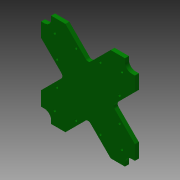
# Autodesk Inventor part: bed2
Saved by Autodesk Inventor 2014 (Build 180170000, 170)
## iProperties
Created: 2015-06-29
Part Number: bed2
Material: Generic
Document SubType Name: Modeling
Designer: cruiser
Density: 1 g/cm^3
Appearance: Default
Author: cruiser
Autodesk Inventor part; units mm, degrees
ref_plane "YZ Plane" through (0, 0, 0) normal (1, 0, 0) x (0, 1, 0)
ref_plane "XZ Plane" through (0, 0, 0) normal (0, 1, 0) x (-1, 0, 0)
ref_plane "XY Plane" through (0, 0, 0) normal (0, 0, 1) x (1, 0, 0)
sketch "Sketch1" plane through (0, 0, 0) normal (0, 1, 0) x (-1, 0, 0)
  line L0 (70.5, -70.5) -> (-70.5, -70.5)
  line L1 (-70.5, -70.5) -> (-70.5, 70.5)
  line L2 (-70.5, 70.5) -> (70.5, 70.5)
  line L3 (70.5, 70.5) -> (70.5, -70.5)
  line L4 (70.5, -70.5) -> (-70.5, 70.5) construction
  line L5 (-70.5, -70.5) -> (70.5, 70.5) construction
  point P0 (0, 0)
  dimension "d0" = 141
  dimension "d1" = 141
  constraints: 12 end point, 2 midpoint, 2 parallel, 1 horizontal, 1 perpendicular
  measures "d0" distance of L1.end L2.end
  measures "d1" distance of L0.end L1.end
extrude "Extrusion1" add sketch "Sketch1" along normal blind 5.88
sketch "Sketch2" plane through (0, 5.88, 0) normal (0, 1, 0) x (1, 0, 0)
  line L0 (75.5, -75.5) -> (-75.5, -75.5)
  line L1 (-75.5, -75.5) -> (-75.5, 75.5)
  line L2 (-75.5, 75.5) -> (75.5, 75.5)
  line L3 (75.5, 75.5) -> (75.5, -75.5)
  line L4 (75.5, -75.5) -> (-75.5, 75.5) construction
  line L5 (-75.5, -75.5) -> (75.5, 75.5) construction
  line L6 (-95.5, 95.5) -> (-55.5, 95.5)
  line L7 (-55.5, 95.5) -> (-55.5, 65.5)
  line L8 (-65.5, 55.5) -> (-95.5, 55.5)
  line L9 (-95.5, 55.5) -> (-95.5, 95.5)
  line L10 (-95.5, 95.5) -> (-55.5, 55.5) construction
  line L11 (-55.5, 95.5) -> (-95.5, 55.5) construction
  arc A0 (-65.5, 55.5) -> (-55.5, 65.5) centre (-65.5, 65.5) ccw
  line L12 (-95.5, -95.5) -> (-55.5, -95.5)
  line L13 (-55.5, -95.5) -> (-55.5, -65.5)
  line L14 (-65.5, -55.5) -> (-95.5, -55.5)
  line L15 (-95.5, -55.5) -> (-95.5, -95.5)
  line L16 (-95.5, -95.5) -> (-55.5, -55.5) construction
  line L17 (-55.5, -95.5) -> (-95.5, -55.5) construction
  arc A1 (-55.5, -65.5) -> (-65.5, -55.5) centre (-65.5, -65.5) ccw
  line L18 (0, 0) -> (0, -75.5)
  line L19 (75.5, -75.5) -> (75.5, 75.5)
  line L20 (95.5, 95.5) -> (55.5, 95.5)
  line L21 (55.5, 95.5) -> (55.5, 65.5)
  line L22 (65.5, 55.5) -> (95.5, 55.5)
  line L23 (95.5, 55.5) -> (95.5, 95.5)
  line L24 (95.5, 95.5) -> (55.5, 55.5) construction
  line L25 (55.5, 95.5) -> (95.5, 55.5) construction
  arc A2 (55.5, 65.5) -> (65.5, 55.5) centre (65.5, 65.5) ccw
  line L26 (95.5, -95.5) -> (55.5, -95.5)
  line L27 (55.5, -95.5) -> (55.5, -65.5)
  line L28 (65.5, -55.5) -> (95.5, -55.5)
  line L29 (95.5, -55.5) -> (95.5, -95.5)
  line L30 (95.5, -95.5) -> (55.5, -55.5) construction
  line L31 (55.5, -95.5) -> (95.5, -55.5) construction
  arc A3 (65.5, -55.5) -> (55.5, -65.5) centre (65.5, -65.5) ccw
  line L32 (70.5, 70.5) -> (70.5, -70.5)
  dimension "d4" = 151
  dimension "d5" = 151
  dimension "d6" = 40
  dimension "d7" = 40
  dimension "d8" = 10
  dimension "d11" = 40
  dimension "d12" = 40
  dimension "d13" = 10
  constraints: 66 end point, 14 symmetric about line, 11 midpoint, 8 point on circle, 8 point on line, 6 parallel, 4 centre point, 4 tangent, 3 horizontal, 3 perpendicular, 2 other
  measures "d4" distance of L1.end L2.end
  measures "d5" distance of L0.end L1.end
  measures "d6" distance of L10.end L8.end
  measures "d7" distance of L6.end L10.end
  measures "d8" radius of A0
  measures "d11" distance of L14.end L16.end
  measures "d12" distance of L16.end L12.end
  measures "d13" radius of A1
extrude "Extrusion2" cut sketch "Sketch2" against normal blind 5.88 contours L3 L28 L29 L26 L27 L0 | L0 L27 A3 L28 L3 | L22 A2 L21 L2 L3 | L3 L2 L21 L20 L23 L22 | L13 L12 L15 L14 L1 L0 | L0 L1 L14 A1 L13 | L7 A0 L8 L1 L2 | L2 L1 L8 L9 L6 L7
sketch "Sketch3" plane through (0, 0, 0) normal (0, -1, 0) x (1, 0, 0)
  line L0 (-55.5, 70.5) -> (-55.5, 65.5) projected
  arc A0 (-65.5, 55.5) -> (-55.5, 65.5) centre (-65.5, 65.5) ccw projected
  line L1 (-65.5, 55.5) -> (-70.5, 55.5) projected
  line L2 (-70.5, 55.5) -> (-70.5, -70.5) projected
  line L3 (-70.5, -70.5) -> (70.5, -70.5) projected
  line L4 (70.5, -70.5) -> (70.5, 70.5) projected
  line L5 (70.5, 70.5) -> (-55.5, 70.5) projected
  point P0 (0, 0)
  point P1 (-60.5, 56.8397)
  constraints: 2 other
extrude "Extrusion3" add sketch "Sketch3" along normal blind 3.15 separate body
sketch "Sketch18" plane through (0, -3.15, 0) normal (0, -1, 0) x (1, 0, 0)
  line L0 (-55.5, 70.5) -> (-55.5, 65.5) projected
  arc A0 (-65.5, 55.5) -> (-55.5, 65.5) centre (-65.5, 65.5) ccw projected
  line L1 (-65.5, 55.5) -> (-70.5, 55.5) projected
  line L2 (-70.5, 55.5) -> (-70.5, -70.5) projected
  line L3 (-70.5, -70.5) -> (70.5, -70.5) projected
  line L4 (70.5, -70.5) -> (70.5, 70.5) projected
  line L5 (70.5, 70.5) -> (-55.5, 70.5) projected
  point P0 (0, 0)
extrude "Extrusion17" add sketch "Sketch18" along normal blind 3.15 separate body
sketch "Sketch5" plane through (0, 5.88, 0) normal (0, 1, 0) x (1, 0, 0)
  line L0 (-55.5, -65.5) -> (-55.5, -70.5) projected
  line L1 (-55.5, -70.5) -> (70.5, -70.5) projected
  line L2 (70.5, -70.5) -> (70.5, 70.5) projected
  line L3 (70.5, 70.5) -> (-70.5, 70.5) projected
  line L4 (-70.5, 70.5) -> (-70.5, -55.5) projected
  line L5 (-70.5, -55.5) -> (-65.5, -55.5) projected
  arc A0 (-55.5, -65.5) -> (-65.5, -55.5) centre (-65.5, -65.5) ccw projected
  point P0 (0, 0)
  point P1 (-60.5, -56.8397)
  constraints: 2 other
extrude "Extrusion5" add sketch "Sketch5" along normal blind 5.88 separate body
sketch "Sketch14" plane through (0, 11.76, 0) normal (0, 1, 0) x (1, 0, 0)
  line L0 (70.5, 70.5) -> (-70.5, 70.5) projected
  line L1 (-70.5, 70.5) -> (-70.5, -55.5) projected
  circle A0 centre (-40.5, 40.5) radius 2
  line L2 (0, 0) -> (10.755, 0)
  line L3 (10.755, 0) -> (10.755, -13.1372)
  line L4 (10.755, -13.1372) -> (0, -13.1372)
  line L5 (0, -13.1372) -> (0, 0)
  circle A1 centre (-50.5, 50.5) radius 1.575
  circle A2 centre (40.5, 40.5) radius 2
  circle A3 centre (50.5, 50.5) radius 1.575
  circle A4 centre (-40.5, -40.5) radius 2
  circle A5 centre (-50.5, -50.5) radius 1.575
  circle A6 centre (40.5, -40.5) radius 2
  circle A7 centre (50.5, -50.5) radius 1.575
  dimension "d87" = 4
  dimension "d88" = 30
  dimension "d89" = 30
  dimension "d90" = 3.15
  dimension "d91" = 20
  dimension "d92" = 20
  constraints: 8 centre point, 8 end point, 6 symmetric about line, 2 parallel, 1 horizontal, 1 perpendicular, 6 other
  measures "d87" diameter of A0
  measures "d88" distance from line of L1 A0.centre
  measures "d89" distance from line of L0 A0.centre
  measures "d90" diameter of A1
  measures "d91" distance from line of L1 A1.centre
  measures "d92" distance from line of L0 A1.centre
extrude "Extrusion14" cut sketch "Sketch14" against normal up to next contours A0 | A1 | A2 | A3 | A4 | A5 | A6 | A7 bodies 4
sketch "Sketch12" plane through (0, 11.76, 0) normal (0, 1, 0) x (1, 0, 0)
  line L0 (70.5, 70.5) -> (-70.5, 70.5) projected
  line L1 (-70.5, 70.5) -> (-70.5, -55.5) projected
  line L2 (0, 20) -> (-50.5, 70.5)
  line L3 (-50.5, 70.5) -> (0, 121)
  line L4 (0, 121) -> (50.5, 70.5)
  line L5 (50.5, 70.5) -> (0, 20)
  line L6 (0, 0) -> (-70.5, 0)
  line L7 (0, 0) -> (0, 70.5)
  line L8 (-20, 0) -> (-70.5, -50.5)
  line L9 (-70.5, -50.5) -> (-121, 0)
  line L10 (-121, 0) -> (-70.5, 50.5)
  line L11 (-70.5, 50.5) -> (-20, 0)
  line L12 (0, -20) -> (-50.5, -70.5)
  line L13 (-50.5, -70.5) -> (0, -121)
  line L14 (0, -121) -> (50.5, -70.5)
  line L15 (50.5, -70.5) -> (0, -20)
  line L16 (20, 0) -> (70.5, -50.5)
  line L17 (70.5, -50.5) -> (121, 0)
  line L18 (121, 0) -> (70.5, 50.5)
  line L19 (70.5, 50.5) -> (20, 0)
  point P0 (-70.5, 0)
  dimension "d76" = 20
  dimension "d77" = 20
  constraints: 36 end point, 8 symmetric about line, 3 point on line, 2 perpendicular, 1 coincident, 1 midpoint, 18 other
  measures "d76" distance of L6.start L2.start
  measures "d77" distance of L6.start L8.start
extrude "Extrusion12" cut sketch "Sketch12" against normal up to next contours L5 L7 L0 | L0 L3 L4 | L7 L2 L0 | L8 L1 L6 | L6 L1 L11 | L1 L9 L10 | L15 L14 L13 L12 | L19 L18 L17 L16 bodies 4
sketch "Sketch15" plane through (0, 5.88, 0) normal (0, 1, 0) x (1, 0, 0)
  line L0 (70.5, 70.5) -> (-70.5, 70.5) projected
  line L1 (-70.5, 70.5) -> (-70.5, -55.5) projected
  circle A0 centre (-50.5, 50.5) radius 2
  circle A1 centre (-40.5, 40.5) radius 4
  line L2 (0, 0) -> (13.8071, 0)
  line L3 (13.8071, 0) -> (13.8071, -11.5249)
  line L4 (13.8071, -11.5249) -> (0, -11.5249)
  line L5 (0, -11.5249) -> (0, 0)
  circle A2 centre (50.5, 50.5) radius 2
  circle A3 centre (40.5, 40.5) radius 4
  circle A4 centre (-50.5, -50.5) radius 2
  circle A5 centre (-40.5, -40.5) radius 4
  circle A6 centre (40.5, -40.5) radius 4
  circle A7 centre (50.5, -50.5) radius 2
  point P0 (-70.5, -55.5)
  point P1 (-60.5, -56.8397)
  dimension "d95" = 8
  dimension "d96" = 4
  dimension "d97" = 30
  dimension "d98" = 30
  dimension "d99" = 20
  dimension "d100" = 20
  constraints: 8 centre point, 8 end point, 6 symmetric about line, 2 parallel, 1 horizontal, 1 perpendicular, 7 other
  measures "d95" diameter of A1
  measures "d96" diameter of A0
  measures "d98" distance from line of L0 A1.centre
  measures "d100" distance from line of L0 A0.centre
extrude "Extrusion15" cut sketch "Sketch15" against normal up to next contours A0 | A2 | A4 | A7 bodies 1
sketch "Sketch9" plane through (0, 5.88, 0) normal (0, 1, 0) x (1, 0, 0)
  line L0 (70.5, -70.5) -> (70.5, 70.5) projected
  line L1 (-70.5, -55.5) -> (-65.5, -55.5) projected
  circle A0 centre (47, 18.28) radius 2
  line L2 (70.5, 30) -> (0, 30)
  line L3 (0, 0) -> (70.5, 70.5)
  circle A1 centre (18.28, 47) radius 2
  dimension "d58" = 4
  dimension "d59" = 47
  dimension "d60" = 30
  dimension "d61" = 11.72
  constraints: 4 end point, 2 centre point, 1 parallel, 1 point on line, 1 symmetric about line, 1 other
  measures "d58" diameter of A0
  measures "d59" horizontal distance of L3.start A0.centre
  measures "d60" distance from line of L3.start L2
  measures "d61" distance from line of L2 A0.centre
extrude "Extrusion9" cut sketch "Sketch9" against normal up to next contours A0 | A1 bodies 1
sketch "Sketch16" plane through (0, 0, 0) normal (0, 1, 0) x (1, 0, 0)
  line L0 (-70.5, 70.5) -> (70.5, 70.5) projected
  circle A0 centre (-50.5, 50.5) radius 4
  line L1 (0, 0) -> (13.4297, 0)
  line L2 (13.4297, 0) -> (13.4297, -12.6623)
  line L3 (13.4297, -12.6623) -> (0, -12.6623)
  line L4 (0, -12.6623) -> (0, 0)
  circle A1 centre (50.5, 50.5) radius 4
  circle A2 centre (-50.5, -50.5) radius 4
  circle A3 centre (50.5, -50.5) radius 4
  point P0 (-70.5, -55.5)
  dimension "d103" = 8
  dimension "d104" = 20
  dimension "d105" = 20
  constraints: 8 end point, 4 centre point, 3 symmetric about line, 2 parallel, 1 horizontal, 1 perpendicular, 4 other
  measures "d103" diameter of A0
  measures "d105" distance from line of L0 A0.centre
extrude "Extrusion16" cut sketch "Sketch16" against normal up to next contours A0 | A1 | A2 | A3 bodies 2
sketch "Sketch19" plane through (0, 11.76, 0) normal (0, 1, 0) x (1, 0, 0)
  line L0 (0, 20) -> (-50.5, 70.5) projected
  line L1 (50.5, 70.5) -> (0, 20) projected
  line L2 (0, 12.9289) -> (-28.2843, 41.2132)
  line L3 (-28.2843, 41.2132) -> (0, 69.4975)
  line L4 (0, 69.4975) -> (28.2843, 41.2132)
  line L5 (28.2843, 41.2132) -> (0, 12.9289)
  line L6 (-12.9289, 0) -> (-41.2132, -28.2843)
  line L7 (-41.2132, -28.2843) -> (-69.4975, 0)
  line L8 (-69.4975, 0) -> (-41.2132, 28.2843)
  line L9 (-41.2132, 28.2843) -> (-12.9289, 0)
  line L10 (0, -12.9289) -> (28.2843, -41.2132)
  line L11 (28.2843, -41.2132) -> (0, -69.4975)
  line L12 (0, -69.4975) -> (-28.2843, -41.2132)
  line L13 (-28.2843, -41.2132) -> (0, -12.9289)
  line L14 (12.9289, 0) -> (41.2132, 28.2843)
  line L15 (41.2132, 28.2843) -> (69.4975, 0)
  line L16 (69.4975, 0) -> (41.2132, -28.2843)
  line L17 (41.2132, -28.2843) -> (12.9289, 0)
  line L18 (-28.2843, 41.2132) -> (28.2843, 41.2132)
  line L19 (28.2843, 41.2132) -> (28.2843, 81.2132)
  line L20 (28.2843, 81.2132) -> (-28.2843, 81.2132)
  line L21 (-28.2843, 81.2132) -> (-28.2843, 41.2132)
  line L22 (-41.2132, -28.2843) -> (-41.2132, 28.2843)
  line L23 (-41.2132, 28.2843) -> (-81.2132, 28.2843)
  line L24 (-81.2132, 28.2843) -> (-81.2132, -28.2843)
  line L25 (-81.2132, -28.2843) -> (-41.2132, -28.2843)
  line L26 (28.2843, -41.2132) -> (-28.2843, -41.2132)
  line L27 (-28.2843, -41.2132) -> (-28.2843, -81.2132)
  line L28 (-28.2843, -81.2132) -> (28.2843, -81.2132)
  line L29 (28.2843, -81.2132) -> (28.2843, -41.2132)
  line L30 (41.2132, 28.2843) -> (41.2132, -28.2843)
  line L31 (41.2132, -28.2843) -> (81.2132, -28.2843)
  line L32 (81.2132, -28.2843) -> (81.2132, 28.2843)
  line L33 (81.2132, 28.2843) -> (41.2132, 28.2843)
  point P0 (0, 0)
  dimension "d110" = 5
  dimension "d111" = 5
  dimension "d112" = 40
  dimension "d113" = 40
  dimension "d116" = 360
  dimension "d127" = 40
  dimension "d130" = 360
  constraints: 64 end point, 5 parallel, 2 perpendicular, 66 other
  measures "d110" distance between parallel lines of L1 L5
  measures "d111" distance between parallel lines of L2 L0
  measures "d112" distance of L2.end L3.end
  measures "d113" distance between parallel lines of L3 L5
  measures "d127" distance of L4.end L19.end
extrude "Extrusion18" cut sketch "Sketch19" against normal up to next bodies 4
sketch "Sketch20" plane through (0, 5.88, 0) normal (0, 1, 0) x (1, 0, 0)
  line L0 (70.5, 70.5) -> (-70.5, 70.5) projected
  line L1 (0, 36.5) -> (-34, 70.5)
  line L2 (-34, 70.5) -> (0, 104.5)
  line L3 (0, 104.5) -> (34, 70.5)
  line L4 (34, 70.5) -> (0, 36.5)
  line L5 (-36.5, 0) -> (-70.5, -34)
  line L6 (-70.5, -34) -> (-104.5, 0)
  line L7 (-104.5, 0) -> (-70.5, 34)
  line L8 (-70.5, 34) -> (-36.5, 0)
  line L9 (0, -36.5) -> (34, -70.5)
  line L10 (34, -70.5) -> (0, -104.5)
  line L11 (0, -104.5) -> (-34, -70.5)
  line L12 (-34, -70.5) -> (0, -36.5)
  line L13 (36.5, 0) -> (70.5, 34)
  line L14 (70.5, 34) -> (104.5, 0)
  line L15 (104.5, 0) -> (70.5, -34)
  line L16 (70.5, -34) -> (36.5, 0)
  point P0 (0, 0)
  point P1 (0, 70.5)
  point P2 (0, 0)
  point P3 (-70.5, 0)
  point P4 (0, 0)
  point P5 (0, -70.5)
  point P6 (0, 0)
  point P7 (70.5, 0)
  dimension "d120" = 34
  dimension "d123" = 360
  constraints: 32 end point, 2 coincident, 1 midpoint, 1 point on line, 48 other
  measures "d120" distance from line of L0 L1.start
extrude "Extrusion19" cut sketch "Sketch20" against normal up to next bodies 1
sketch "Sketch23" plane through (0, 11.76, 0) normal (0, 1, 0) x (1, 0, 0)
  line L0 (-75.5, -75.5) -> (75.5, -75.5)
  line L1 (75.5, -75.5) -> (75.5, 75.5)
  line L2 (75.5, 75.5) -> (-75.5, 75.5)
  line L3 (-75.5, 75.5) -> (-75.5, -75.5)
  line L4 (-75.5, -75.5) -> (75.5, 75.5) construction
  line L5 (75.5, -75.5) -> (-75.5, 75.5) construction
  line L6 (-70.5, 55.5) -> (-95.5, 55.5)
  line L7 (-95.5, 55.5) -> (-95.5, 95.5)
  line L8 (-95.5, 95.5) -> (-55.5, 95.5)
  line L9 (-55.5, 95.5) -> (-55.5, 70.5)
  line L10 (-55.5, 55.5) -> (-95.5, 95.5) construction
  line L11 (-95.5, 55.5) -> (-55.5, 95.5) construction
  arc A0 (-70.5, 55.5) -> (-55.5, 70.5) centre (-70.5, 70.5) ccw
  line L12 (-55.5, -70.5) -> (-55.5, -95.5)
  line L13 (-55.5, -95.5) -> (-95.5, -95.5)
  line L14 (-95.5, -95.5) -> (-95.5, -55.5)
  line L15 (-95.5, -55.5) -> (-70.5, -55.5)
  line L16 (-55.5, -55.5) -> (-95.5, -95.5) construction
  line L17 (-55.5, -95.5) -> (-95.5, -55.5) construction
  arc A1 (-55.5, -70.5) -> (-70.5, -55.5) centre (-70.5, -70.5) ccw
  line L18 (70.5, -55.5) -> (95.5, -55.5)
  line L19 (95.5, -55.5) -> (95.5, -95.5)
  line L20 (95.5, -95.5) -> (55.5, -95.5)
  line L21 (55.5, -95.5) -> (55.5, -70.5)
  line L22 (55.5, -55.5) -> (95.5, -95.5) construction
  line L23 (95.5, -55.5) -> (55.5, -95.5) construction
  arc A2 (70.5, -55.5) -> (55.5, -70.5) centre (70.5, -70.5) ccw
  line L24 (55.5, 70.5) -> (55.5, 95.5)
  line L25 (55.5, 95.5) -> (95.5, 95.5)
  line L26 (95.5, 95.5) -> (95.5, 55.5)
  line L27 (95.5, 55.5) -> (70.5, 55.5)
  line L28 (55.5, 55.5) -> (95.5, 95.5) construction
  line L29 (55.5, 95.5) -> (95.5, 55.5) construction
  arc A3 (55.5, 70.5) -> (70.5, 55.5) centre (70.5, 70.5) ccw
  point P0 (-70.5, 70.5)
  point P1 (-70.5, 50.5)
  point P2 (0, 0)
  point P3 (-70.5, -70.5)
  point P4 (-50.5, -70.5)
  point P5 (-75.5, -75.5)
  point P6 (70.5, -70.5)
  point P7 (70.5, -50.5)
  point P8 (75.5, -75.5)
  point P9 (70.5, 70.5)
  point P10 (50.5, 70.5)
  point P11 (75.5, 75.5)
  dimension "d135" = 151
  dimension "d136" = 151
  dimension "d137" = 40
  dimension "d138" = 40
  dimension "d139" = 15
  dimension "d142" = 360
  constraints: 60 end point, 10 midpoint, 8 point on circle, 8 point on line, 4 centre point, 4 parallel, 2 horizontal, 2 perpendicular, 2 tangent, 69 other
  measures "d135" distance of L2.end L1.end
  measures "d136" distance of L1.end L0.end
  measures "d137" distance of L7.end L8.end
  measures "d138" distance of L6.end L7.end
  measures "d139" radius of A0
extrude "Extrusion20" cut sketch "Sketch23" against normal up to next contours L21 A2 L18 L1 L0 | L0 L1 L18 L19 L20 L21 | L6 L7 L8 L9 L2 L3 | L3 L2 L9 A0 L6 | L27 A3 L24 L2 L1 | L1 L2 L24 L25 L26 L27 bodies 4
fillet "Fillet1" radius 5 8 edges at (36.5, 2.94, 0) (0, 2.94, -36.5) (-36.5, 2.94, 0) (0, 2.94, 36.5) (0, 8.82, -12.9289) (12.9289, 8.82, 0) (0, 8.82, 12.9289) (-12.9289, 8.82, 0)
pattern_circular "Circular Pattern1" count 4 over 360 about axis through (0, -10, 0) along (0, 1, 0) of "Extrusion9" bodies 1
equation "\"d0\" = bed_x"
equation "\"d1\" = bed_y"
equation "\"d2\" = t_wall"
equation "\"d4\" = reservoir_x"
equation "\"d5\" = reservoir_y"
equation "\"d9\" = t_wall"
equation "\"d14\" = clear_acrylic"
equation "\"d108\" = thin_acrylic"
equation "\"d18\" = t_carrier"
equation "\"d87\" = brass_insert_drill"
equation "\"d88\" = spring_border"
equation "\"d89\" = spring_border"
equation "\"d90\" = m3_diameter"
equation "\"d91\" = bed_clamp_border"
equation "\"d92\" = bed_clamp_border"
equation "\"d96\" = brass_insert_drill"
equation "\"d97\" = spring_border"
equation "\"d98\" = spring_border"
equation "\"d99\" = bed_clamp_border"
equation "\"d100\" = bed_clamp_border"
equation "\"d101\" = t_carrier"
equation "\"d58\" = brass_insert_drill"
equation "\"d59\" = end_stop_offset_x"
equation "\"d60\" = 0.5 * crane_y"
equation "\"d61\" = thumb_nut_offset_y"
equation "\"d104\" = bed_clamp_border"
equation "\"d105\" = bed_clamp_border"
equation "\"d106\" = t_carrier"
equation "\"thick_acrylic\" = 5.88"
equation "\"thin_acrylic\" = 3.15"
equation "\"clear_acrylic\" = 3.15"
equation "\"wood_thickness\" = 6.72"
equation "\"m3_diameter\" = 3.15"
equation "\"m4_diameter\" = 4.2"
equation "\"m5_diameter\" = 5.25"
equation "\"brass_insert_drill\" = 4"
equation "\"stepper_screw_space\" = 35"
equation "\"stepper_shaft_diameter\" = 5"
equation "\"stepper_body_diameter\" = 28"
equation "\"laser_body_diameter\" = 12"
equation "\"t_carrier\" = 5.88"
equation "\"t_wall\" = 5.88"
equation "\"t_window\" = 3.15"
equation "\"carrier_y\" = 181"
equation "\"carrier_z\" = 258.04"
equation "\"carrier_z2\" = 283.04"
equation "\"window_z\" = 185"
equation "\"window_y\" = 49.56"
equation "\"reservoir_x\" = 151"
equation "\"reservoir_y\" = 151"
equation "\"linear_bearing_spacing\" = 207"
equation "\"linear_bearing_z\" = 304.8"
equation "\"threaded_rod_z\" = 203.2"
equation "\"motor_spacing\" = 287"
equation "\"t_tray\" = 3.15"
equation "\"tray_border\" = 15"
equation "\"tray_x\" = 181"
equation "\"tray_y\" = 181"
equation "\"bed_x\" = 141"
equation "\"bed_y\" = 141"
equation "\"spring_border\" = 30"
equation "\"bed_clamp_border\" = 20"
equation "\"brass_keep_out\" = 8"
equation "\"tape_keep_out\" = 2"
equation "\"tape_thickness\" = 2"
equation "\"crane_x\" = 244.56"
equation "\"crane_z\" = 25"
equation "\"z_min_from_center\" = 72.28"
equation "\"t_frame\" = 6.72"
equation "\"frame_top_z\" = 295"
equation "\"frame_bottom_z\" = 225"
equation "\"frame_y\" = 68.44"
equation "\"frame_border\" = 39.5"
equation "\"frame_tilt\" = 1deg"
equation "\"printer_z\" = 289"
equation "\"lcd_x\" = 72"
equation "\"lcd_y\" = 25"
equation "\"subframe_y_offset\" = 27.5"
equation "\"laser_y_offset\" = 19.4"
equation "\"laser_diameter\" = 12"
equation "\"laser_z_offset\" = 55"
equation "\"laser_y\" = 35"
equation "\"laser_z\" = 18"
equation "\"t_galvo_frame\" = 6.72"
equation "\"galvo_frame_x\" = 66"
equation "\"galvo_frame_z\" = 65"
equation "\"galvo_frame_y_offset\" = 27.5"
equation "\"laser_x\" = 24"
equation "\"drawer_z\" = 206.72"
equation "\"drawer_y\" = 49.56"
equation "\"drawer_x\" = 181"
equation "\"frame_foot_z\" = 49.5"
equation "\"drawer_z_from_bottom\" = 25"
equation "\"end_stop_offset_x\" = 47"
equation "\"t_crane\" = 6.72"
equation "\"end_stop_spacing\" = 19"
equation "\"thumb_nut_offset_y\" = 11.72"
equation "\"thumb_nut_diameter\" = 7"
equation "\"frame_foot_extension\" = 4"
equation "\"m5_brass_insert_drill\" = 6.7"
equation "\"m3_brass_insert_drill\" = 4"
equation "\"door_sensor\" = 35"
equation "\"protection_slot_offset\" = 45.25"
equation "\"protection_slot\" = 36.2"
equation "\"protection_slot_length\" = 35"
equation "\"m3_main_nut_width\" = 5.7"
equation "\"m3_main_length\" = 14"
equation "\"m3_main_extra\" = 1"
equation "\"m3_main_nut_thickness\" = 2.5"
equation "\"crane_y\" = 60"
